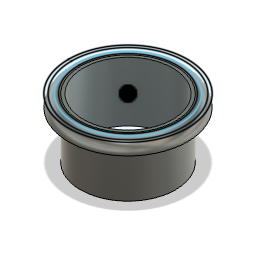
button_holder (Autodesk Fusion 360 design; units mm, degrees)
Autodesk Fusion 360 part; units mm, degrees
sketch "Sketch1" plane through (0, 0, 0) normal (0, 1, 0) x (1, 0, 0)
  circle A0 centre (0, 0) radius 15
  circle A1 centre (0, 0) radius 17.5
  dimension "d1" = 30
  dimension "d2" = 35
  constraint coincident A0.centre A1.centre
  measures "d1" diameter of A0
  measures "d2" diameter of A1
extrude "Extrude1" add sketch "Sketch1" along normal blind 20
sketch "Sketch2" plane through (0, 20, 0) normal (0, 1, 0) x (-1, 0, 0)
  circle A0 centre (0, 0) radius 15
  circle A1 centre (0, 0) radius 17.5
  circle A2 centre (0, 0) radius 16.5
  circle A3 centre (0, 0) radius 17.5
  circle A4 centre (0, 0) radius 19
  circle A5 centre (0, 0) radius 20
  dimension "d5" = 33
  dimension "d10" = 38
  dimension "d13" = 40
  constraint coincident A0.centre A1.centre
  constraint concentric A3 A4
  constraint concentric A4 A5
  measures "d5" diameter of A2
  measures "d10" diameter of A4
  measures "d13" diameter of A5
extrude "Extrude2" cut sketch "Sketch2" against normal blind 20 contours A1 A3
extrude "Extrude3" add sketch "Sketch2" against normal blind 2 contours A1 A3
extrude "Extrude4" add sketch "Sketch2" against normal blind 4 contours A1 A3 | A4
extrude "Extrude5" add sketch "Sketch2" against normal blind 4 contours A5
sketch "Sketch3" plane through (0, 0, 0) normal (0, -1, 0) x (1, 0, 0)
  circle A0 centre (0, 0) radius 16.5
  circle A1 centre (0, 0) radius 15
  circle A2 centre (0, 0) radius 16
  circle A3 centre (0, 0) radius 16.5
  constraint coincident A0.centre A1.centre
extrude "Extrude6" cut sketch "Sketch3" against normal blind 16 contours A0 A3
fillet "Fillet1" radius 4 1 edges at (18.6465, 20, -7.2323)
